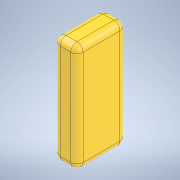
# Autodesk Inventor part: Battery
Saved by Autodesk Inventor 2021 (Build 250183000, 183)
## iProperties
Created: 2024-02-01
Part Number: Battery
Material: Generic
Document SubType Name: Modeling
Designer: maxsm
Density: 1 g/cm^3
Appearance: Default
Author: maxsm
Autodesk Inventor part; units mm, degrees
ref_plane "YZ Plane" through (0, 0, 0) normal (1, 0, 0) x (0, 1, 0)
ref_plane "XZ Plane" through (0, 0, 0) normal (0, 1, 0) x (-1, 0, 0)
ref_plane "XY Plane" through (0, 0, 0) normal (0, 0, 1) x (1, 0, 0)
sketch "Sketch1" plane through (0, 0, 0) normal (0, 1, 0) x (-1, 0, 0)
  line L0 (3.75, 8) -> (-3.75, 8)
  line L1 (-3.75, 8) -> (-3.75, -8)
  line L2 (-3.75, -8) -> (3.75, -8)
  line L3 (3.75, -8) -> (3.75, 8)
  line L4 (3.75, 8) -> (-3.75, -8) construction
  line L5 (-3.75, 8) -> (3.75, -8) construction
  point P0 (0, 0)
  dimension "d0" = 7.5
  dimension "d1" = 16
  constraints: 12 end point, 2 midpoint, 2 parallel, 1 horizontal, 1 perpendicular
  measures "d0" distance of L2.end L1.end
  measures "d1" distance of L1.end L0.end
extrude "Extrusion1" add sketch "Sketch1" along normal blind 35
fillet "Fillet1" radius 2 12 edges at (3.75, 17.5, 8) (3.75, 35, 0) (-3.75, 35, 0) (0, 35, 8) (-3.75, 17.5, 8) (3.75, 17.5, -8) (0, 35, -8) (-3.75, 17.5, -8) (0, 0, -8) (-3.75, 0, 0) (0, 0, 8) (3.75, 0, 0)
body "Solid1"
